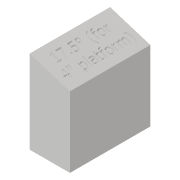
# Autodesk Inventor part: 20DegreeStand
Saved by Autodesk Inventor 2018 (Build 220112000, 112)
## iProperties
Created: 2018-12-13
Part Number: 20DegreeStand
Material: Generic
Document SubType Name: Modeling
Designer: ball
Density: 1 g/cm^3
Appearance: Default
Author: ball
Autodesk Inventor part; units mm, degrees
ref_plane "YZ Plane" through (0, 0, 0) normal (1, 0, 0) x (0, 1, 0)
ref_plane "XZ Plane" through (0, 0, 0) normal (0, 1, 0) x (-1, 0, 0)
ref_plane "XY Plane" through (0, 0, 0) normal (0, 0, 1) x (1, 0, 0)
sketch "Sketch1" plane through (0, 0, 0) normal (0, 1, 0) x (-1, 0, 0)
  line L0 (0, 0) -> (12.7, 0)
  line L1 (12.7, 0) -> (12.7, -25.4)
  line L2 (12.7, -25.4) -> (0, -25.4)
  line L3 (0, -25.4) -> (0, 0)
  dimension "d0" = 12.7
  dimension "d1" = 25.4
  constraints: 8 end point, 2 parallel, 1 horizontal, 1 perpendicular
  measures "d0" distance of L1.end L2.end
  measures "d1" distance of L0.end L1.end
extrude "Extrusion1" add sketch "Sketch1" along normal blind 26.289
sketch "Sketch2" plane through (-12.7, 0, 0) normal (0, 0, 1) x (1, 0, 0)
  line L0 (0, 0) -> (0, 26.289) projected
  line L1 (0, 26.289) -> (12.7, 26.289) projected
  line L2 (0, 26.289) -> (12.7, 26.289)
  line L3 (0, 26.289) -> (12.7, 22.2847)
  line L4 (0, 26.289) -> (13.3163, 26.289) construction
  line L5 (12.7, 0) -> (12.7, 26.289) projected
  line L6 (12.7, 22.2847) -> (12.7, 26.289)
  dimension "d4" = 17.5
  constraints: 8 end point, 1 collinear, 1 equal length, 1 horizontal, 1 perpendicular
  measures "d4" angle of L3 L4
extrude "Extrusion2" cut sketch "Sketch2" against normal blind 26.289
sketch "Sketch3" plane through (-12.7, 26.289, 0) normal (0.3007058, 0.953717, 0) x (0.953717, -0.3007058, 0)
  line L0 (2.3231, -6.9377) -> (2.3231, 32.6962) construction
  line L1 (2.3231, 32.6962) -> (11.3899, 32.6962) construction
  line L2 (11.3899, 32.6962) -> (11.3899, -6.9377) construction
  line L3 (11.3899, -6.9377) -> (2.3231, -6.9377) construction
  line L4 (5.5267, 5.1037) -> (5.5267, 3.6167)
  line L5 (5.5267, 3.6167) -> (5.2155, 3.6167)
  line L6 (5.2155, 3.6167) -> (5.2155, 4.17)
  line L7 (5.2155, 4.17) -> (3.1727, 4.17)
  line L8 (3.1727, 4.17) -> (3.1727, 3.6167)
  line L9 (3.1727, 3.6167) -> (2.8936, 3.6167)
  spline S0 degree 2 poles (2.8936, 3.6167) (2.8936, 3.9304) (2.7158, 4.2268) (2.4688, 4.2466) knots 0 0 0 1 2 2 2
  line L10 (2.4688, 4.2466) -> (2.4688, 4.5627)
  line L11 (2.4688, 4.5627) -> (5.2155, 4.5627)
  line L12 (5.2155, 4.5627) -> (5.2155, 5.1037)
  line L13 (5.2155, 5.1037) -> (5.5267, 5.1037)
  line L14 (2.9356, 7.5786) -> (5.5267, 6.2596)
  line L15 (5.5267, 6.2596) -> (5.5267, 5.8249)
  line L16 (5.5267, 5.8249) -> (2.8368, 7.218)
  line L17 (2.8368, 7.218) -> (2.8368, 5.6446)
  line L18 (2.8368, 5.6446) -> (2.4787, 5.6446)
  line L19 (2.4787, 5.6446) -> (2.4787, 7.5786)
  line L20 (2.4787, 7.5786) -> (2.9356, 7.5786)
  line L21 (5.5267, 8.6061) -> (5.5267, 8.1171)
  line L22 (5.5267, 8.1171) -> (4.9437, 8.1171)
  line L23 (4.9437, 8.1171) -> (4.9437, 8.6061)
  line L24 (4.9437, 8.6061) -> (5.5267, 8.6061)
  spline S1 degree 2 poles (4.5584, 11.0687) (4.7783, 11.0687) (5.1537, 10.928) (5.292, 10.7995) knots 0 0 0 1 2 2 2
  spline S2 degree 2 poles (5.292, 10.7995) (5.4303, 10.6711) (5.5909, 10.2882) (5.5909, 10.0511) knots 0 0 0 1 2 2 2
  spline S3 degree 2 poles (5.5909, 10.0511) (5.5909, 9.8337) (5.4946, 9.4089) (5.418, 9.2533) knots 0 0 0 1 2 2 2
  line L25 (5.418, 9.2533) -> (4.9857, 9.2533)
  line L26 (4.9857, 9.2533) -> (4.9857, 9.2829)
  spline S4 degree 2 poles (4.9857, 9.2829) (5.0203, 9.3299) (5.1092, 9.5052) (5.1488, 9.6114) knots 0 0 0 1 2 2 2
  spline S5 degree 2 poles (5.1488, 9.6114) (5.1907, 9.7325) (5.2377, 9.9325) (5.2377, 10.0585) knots 0 0 0 1 2 2 2
  spline S6 degree 2 poles (5.2377, 10.0585) (5.2377, 10.182) (5.1488, 10.4142) (5.0524, 10.4982) knots 0 0 0 1 2 2 2
  spline S7 degree 2 poles (5.0524, 10.4982) (4.961, 10.5747) (4.719, 10.6538) (4.556, 10.6538) knots 0 0 0 1 2 2 2
  spline S8 degree 2 poles (4.556, 10.6538) (4.3929, 10.6538) (4.1855, 10.5649) (4.1163, 10.4809) knots 0 0 0 1 2 2 2
  spline S9 degree 2 poles (4.1163, 10.4809) (4.0397, 10.3944) (3.9755, 10.1376) (3.9755, 9.9819) knots 0 0 0 1 2 2 2
  spline S10 degree 2 poles (3.9755, 9.9819) (3.9755, 9.814) (4.0274, 9.4805) (4.0496, 9.3793) knots 0 0 0 1 2 2 2
  line L27 (4.0496, 9.3793) -> (2.4787, 9.3793)
  line L28 (2.4787, 9.3793) -> (2.4787, 11.0515)
  line L29 (2.4787, 11.0515) -> (2.8368, 11.0515)
  line L30 (2.8368, 11.0515) -> (2.8368, 9.772)
  line L31 (2.8368, 9.772) -> (3.6495, 9.772)
  spline S11 degree 2 poles (3.6495, 9.772) (3.6396, 9.8461) (3.6322, 9.9894) (3.6322, 10.0486) knots 0 0 0 1 2 2 2
  spline S12 degree 2 poles (3.6322, 10.0486) (3.6322, 10.2833) (3.7087, 10.6069) (3.8224, 10.7551) knots 0 0 0 1 2 2 2
  spline S13 degree 2 poles (3.8224, 10.7551) (3.936, 10.9057) (4.2818, 11.0687) (4.5584, 11.0687) knots 0 0 0 1 2 2 2
  spline S14 degree 2 poles (3.2049, 13.0522) (3.5334, 13.0522) (3.9829, 12.6026) (3.9829, 12.2741) knots 0 0 0 1 2 2 2
  spline S15 degree 2 poles (3.9829, 12.2741) (3.9829, 11.9481) (3.5358, 11.4936) (3.2049, 11.4936) knots 0 0 0 1 2 2 2
  spline S16 degree 2 poles (3.2049, 11.4936) (2.8763, 11.4936) (2.4268, 11.9431) (2.4268, 12.2741) knots 0 0 0 1 2 2 2
  spline S17 degree 2 poles (2.4268, 12.2741) (2.4268, 12.6026) (2.8763, 13.0522) (3.2049, 13.0522) knots 0 0 0 1 2 2 2
  spline S18 degree 2 poles (3.2049, 12.7311) (3.0073, 12.7311) (2.738, 12.4692) (2.738, 12.2741) knots 0 0 0 1 2 2 2
  spline S19 degree 2 poles (2.738, 12.2741) (2.738, 12.0765) (3.0073, 11.8147) (3.2049, 11.8147) knots 0 0 0 1 2 2 2
  spline S20 degree 2 poles (3.2049, 11.8147) (3.4049, 11.8147) (3.6717, 12.0815) (3.6717, 12.2741) knots 0 0 0 1 2 2 2
  spline S21 degree 2 poles (3.6717, 12.2741) (3.6717, 12.4692) (3.4, 12.7311) (3.2049, 12.7311) knots 0 0 0 1 2 2 2
  line L32 (6.3689, 16.0211) -> (6.3689, 15.5518)
  spline S22 degree 2 poles (6.3689, 15.5518) (5.9466, 15.1961) (5.0006, 14.7886) (4.3559, 14.7886) knots 0 0 0 1 2 2 2
  spline S23 degree 2 poles (4.3559, 14.7886) (3.726, 14.7886) (2.7652, 15.1912) (2.3428, 15.5518) knots 0 0 0 1 2 2 2
  line L33 (2.3428, 15.5518) -> (2.3428, 16.0211)
  line L34 (2.3428, 16.0211) -> (2.3626, 16.0211)
  spline S24 degree 2 poles (2.3626, 16.0211) (2.5133, 15.8556) (2.9035, 15.5543) (3.1629, 15.4259) knots 0 0 0 1 2 2 2
  spline S25 degree 2 poles (3.1629, 15.4259) (3.4148, 15.3024) (4.02, 15.1492) (4.3559, 15.1492) knots 0 0 0 1 2 2 2
  spline S26 degree 2 poles (4.3559, 15.1492) (4.7066, 15.1492) (5.2871, 15.2974) (5.5489, 15.4259) knots 0 0 0 1 2 2 2
  spline S27 degree 2 poles (5.5489, 15.4259) (5.8008, 15.5494) (6.2084, 15.863) (6.3492, 16.0211) knots 0 0 0 1 2 2 2
  line L35 (6.3492, 16.0211) -> (6.3689, 16.0211)
  line L36 (2.7133, 17.6563) -> (2.7133, 17.6365)
  spline S28 degree 2 poles (2.7133, 17.6365) (2.6936, 17.5847) (2.659, 17.392) (2.659, 17.3154) knots 0 0 0 1 2 2 2
  spline S29 degree 2 poles (2.659, 17.3154) (2.659, 17.0734) (2.8763, 16.8659) (3.1629, 16.8659) knots 0 0 0 1 2 2 2
  line L37 (3.1629, 16.8659) -> (3.2394, 16.8659)
  line L38 (3.2394, 16.8659) -> (3.2394, 17.5031)
  line L39 (3.2394, 17.5031) -> (3.5581, 17.5031)
  line L40 (3.5581, 17.5031) -> (3.5581, 16.8782)
  line L41 (3.5581, 16.8782) -> (5.5267, 16.8782)
  line L42 (5.5267, 16.8782) -> (5.5267, 16.4929)
  line L43 (5.5267, 16.4929) -> (3.5581, 16.4929)
  line L44 (3.5581, 16.4929) -> (3.5581, 16.2336)
  line L45 (3.5581, 16.2336) -> (3.2394, 16.2336)
  line L46 (3.2394, 16.2336) -> (3.2394, 16.4929)
  line L47 (3.2394, 16.4929) -> (3.1629, 16.4929)
  spline S30 degree 2 poles (3.1629, 16.4929) (2.7528, 16.4929) (2.3231, 16.8906) (2.3231, 17.2611) knots 0 0 0 1 2 2 2
  spline S31 degree 2 poles (2.3231, 17.2611) (2.3231, 17.3673) (2.3453, 17.5723) (2.3601, 17.6563) knots 0 0 0 1 2 2 2
  line L48 (2.3601, 17.6563) -> (2.7133, 17.6563)
  spline S32 degree 2 poles (4.3831, 19.6669) (4.961, 19.6669) (5.5909, 19.1111) (5.5909, 18.6468) knots 0 0 0 1 2 2 2
  spline S33 degree 2 poles (5.5909, 18.6468) (5.5909, 18.17) (4.9413, 17.6242) (4.3831, 17.6242) knots 0 0 0 1 2 2 2
  spline S34 degree 2 poles (4.3831, 17.6242) (3.81, 17.6242) (3.1752, 18.1873) (3.1752, 18.6468) knots 0 0 0 1 2 2 2
  spline S35 degree 2 poles (3.1752, 18.6468) (3.1752, 19.1111) (3.8075, 19.6669) (4.3831, 19.6669) knots 0 0 0 1 2 2 2
  spline S36 degree 2 poles (4.3831, 19.2692) (3.9385, 19.2692) (3.5062, 18.9456) (3.5062, 18.6468) knots 0 0 0 1 2 2 2
  spline S37 degree 2 poles (3.5062, 18.6468) (3.5062, 18.3479) (3.9385, 18.0218) (4.3831, 18.0218) knots 0 0 0 1 2 2 2
  spline S38 degree 2 poles (4.3831, 18.0218) (4.8153, 18.0218) (5.2599, 18.3479) (5.2599, 18.6468) knots 0 0 0 1 2 2 2
  spline S39 degree 2 poles (5.2599, 18.6468) (5.2599, 18.9432) (4.8227, 19.2692) (4.3831, 19.2692) knots 0 0 0 1 2 2 2
  line L49 (3.6519, 21.2749) -> (3.6519, 21.2551)
  spline S40 degree 2 poles (3.6519, 21.2551) (3.6396, 21.2106) (3.6346, 21.1143) (3.6346, 21.0476) knots 0 0 0 1 2 2 2
  spline S41 degree 2 poles (3.6346, 21.0476) (3.6346, 20.892) (3.7705, 20.5857) (3.9039, 20.4474) knots 0 0 0 1 2 2 2
  line L50 (3.9039, 20.4474) -> (5.5267, 20.4474)
  line L51 (5.5267, 20.4474) -> (5.5267, 20.0621)
  line L52 (5.5267, 20.0621) -> (3.2394, 20.0621)
  line L53 (3.2394, 20.0621) -> (3.2394, 20.4474)
  line L54 (3.2394, 20.4474) -> (3.5803, 20.4474)
  spline S42 degree 2 poles (3.5803, 20.4474) (3.3926, 20.6574) (3.2394, 20.971) (3.2394, 21.1192) knots 0 0 0 1 2 2 2
  spline S43 degree 2 poles (3.2394, 21.1192) (3.2394, 21.1785) (3.2444, 21.2378) (3.2518, 21.2749) knots 0 0 0 1 2 2 2
  line L55 (3.2518, 21.2749) -> (3.6519, 21.2749)
  line L56 (9.4978, 3.8612) -> (9.4978, 3.4981)
  line L57 (9.4978, 3.4981) -> (10.5451, 3.4981)
  line L58 (10.5451, 3.4981) -> (10.5451, 3.1054)
  line L59 (10.5451, 3.1054) -> (9.4978, 3.1054)
  line L60 (9.4978, 3.1054) -> (9.4978, 1.7593)
  line L61 (9.4978, 1.7593) -> (9.0681, 1.7593)
  line L62 (9.0681, 1.7593) -> (7.4971, 3.1227)
  line L63 (7.4971, 3.1227) -> (7.4971, 3.4981)
  line L64 (7.4971, 3.4981) -> (9.1693, 3.4981)
  line L65 (9.1693, 3.4981) -> (9.1693, 3.8612)
  line L66 (9.1693, 3.8612) -> (9.4978, 3.8612)
  line L67 (9.1693, 3.1054) -> (7.9788, 3.1054)
  line L68 (7.9788, 3.1054) -> (9.1693, 2.0804)
  line L69 (9.1693, 2.0804) -> (9.1693, 3.1054)
  line L70 (7.3613, 4.6442) -> (8.5469, 4.5553)
  line L71 (8.5469, 4.5553) -> (8.5469, 4.2861)
  line L72 (8.5469, 4.2861) -> (7.3613, 4.1972)
  line L73 (7.3613, 4.1972) -> (7.3613, 4.6442)
  line L74 (7.3613, 5.4149) -> (8.5469, 5.326)
  line L75 (8.5469, 5.326) -> (8.5469, 5.0567)
  line L76 (8.5469, 5.0567) -> (7.3613, 4.9678)
  line L77 (7.3613, 4.9678) -> (7.3613, 5.4149)
  spline S44 degree 2 poles (9.3398, 9.152) (9.9128, 9.152) (10.5896, 8.6061) (10.5896, 8.1887) knots 0 0 0 1 2 2 2
  spline S45 degree 2 poles (10.5896, 8.1887) (10.5896, 8.0183) (10.5105, 7.7565) (10.429, 7.6206) knots 0 0 0 1 2 2 2
  line L78 (10.429, 7.6206) -> (11.3874, 7.6206)
  line L79 (11.3874, 7.6206) -> (11.3874, 7.2353)
  line L80 (11.3874, 7.2353) -> (8.2579, 7.2353)
  line L81 (8.2579, 7.2353) -> (8.2579, 7.6206)
  line L82 (8.2579, 7.6206) -> (8.4975, 7.6206)
  spline S46 degree 2 poles (8.4975, 7.6206) (8.3666, 7.7639) (8.1937, 8.1146) (8.1937, 8.3196) knots 0 0 0 1 2 2 2
  spline S47 degree 2 poles (8.1937, 8.3196) (8.1937, 8.7124) (8.8161, 9.152) (9.3398, 9.152) knots 0 0 0 1 2 2 2
  spline S48 degree 2 poles (9.3842, 8.7543) (8.9915, 8.7543) (8.5592, 8.5049) (8.5592, 8.2258) knots 0 0 0 1 2 2 2
  spline S49 degree 2 poles (8.5592, 8.2258) (8.5592, 8.0627) (8.705, 7.7565) (8.8186, 7.6206) knots 0 0 0 1 2 2 2
  line L83 (8.8186, 7.6206) -> (10.1178, 7.6206)
  spline S50 degree 2 poles (10.1178, 7.6206) (10.1894, 7.7713) (10.2438, 7.9862) (10.2438, 8.1245) knots 0 0 0 1 2 2 2
  spline S51 degree 2 poles (10.2438, 8.1245) (10.2438, 8.4234) (9.8041, 8.7543) (9.3842, 8.7543) knots 0 0 0 1 2 2 2
  line L84 (10.5451, 9.9449) -> (10.5451, 9.5596)
  line L85 (10.5451, 9.5596) -> (7.3613, 9.5596)
  line L86 (7.3613, 9.5596) -> (7.3613, 9.9449)
  line L87 (7.3613, 9.9449) -> (10.5451, 9.9449)
  spline S52 degree 2 poles (10.3031, 11.7851) (10.3376, 11.7381) (10.4611, 11.58) (10.4982, 11.5059) knots 0 0 0 1 2 2 2
  spline S53 degree 2 poles (10.4982, 11.5059) (10.5525, 11.4047) (10.6093, 11.2145) (10.6093, 11.0416) knots 0 0 0 1 2 2 2
  spline S54 degree 2 poles (10.6093, 11.0416) (10.6093, 10.9008) (10.5031, 10.6464) (10.4068, 10.55) knots 0 0 0 1 2 2 2
  spline S55 degree 2 poles (10.4068, 10.55) (10.3129, 10.4587) (10.0363, 10.3475) (9.8832, 10.3475) knots 0 0 0 1 2 2 2
  spline S56 degree 2 poles (9.8832, 10.3475) (9.646, 10.3475) (9.3101, 10.5476) (9.2138, 10.7649) knots 0 0 0 1 2 2 2
  spline S57 degree 2 poles (9.2138, 10.7649) (9.1249, 10.9576) (9.0582, 11.4812) (9.0409, 11.7851) knots 0 0 0 1 2 2 2
  line L88 (9.0409, 11.7851) -> (8.9668, 11.7851)
  spline S58 degree 2 poles (8.9668, 11.7851) (8.8334, 11.7851) (8.6679, 11.7035) (8.621, 11.6294) knots 0 0 0 1 2 2 2
  spline S59 degree 2 poles (8.621, 11.6294) (8.5741, 11.5553) (8.5444, 11.3429) (8.5444, 11.2293) knots 0 0 0 1 2 2 2
  spline S60 degree 2 poles (8.5444, 11.2293) (8.5444, 11.0959) (8.6235, 10.7353) (8.7, 10.555) knots 0 0 0 1 2 2 2
  line L89 (8.7, 10.555) -> (8.7, 10.5328)
  line L90 (8.7, 10.5328) -> (8.3073, 10.5328)
  spline S61 degree 2 poles (8.3073, 10.5328) (8.2776, 10.639) (8.2035, 11.0366) (8.2035, 11.2318) knots 0 0 0 1 2 2 2
  spline S62 degree 2 poles (8.2035, 11.2318) (8.2035, 11.4689) (8.2776, 11.7925) (8.374, 11.9209) knots 0 0 0 1 2 2 2
  spline S63 degree 2 poles (8.374, 11.9209) (8.4678, 12.0469) (8.7667, 12.1704) (8.9816, 12.1704) knots 0 0 0 1 2 2 2
  line L91 (8.9816, 12.1704) -> (10.5451, 12.1704)
  line L92 (10.5451, 12.1704) -> (10.5451, 11.7851)
  line L93 (10.5451, 11.7851) -> (10.3031, 11.7851)
  line L94 (9.982, 11.7851) -> (9.3472, 11.7851)
  spline S64 degree 2 poles (9.3472, 11.7851) (9.3595, 11.6467) (9.4015, 11.2293) (9.441, 11.0984) knots 0 0 0 1 2 2 2
  spline S65 degree 2 poles (9.441, 11.0984) (9.488, 10.9452) (9.6831, 10.7452) (9.856, 10.7452) knots 0 0 0 1 2 2 2
  spline S66 degree 2 poles (9.856, 10.7452) (10.0536, 10.7452) (10.2537, 10.9675) (10.2537, 11.1799) knots 0 0 0 1 2 2 2
  spline S67 degree 2 poles (10.2537, 11.1799) (10.2537, 11.3602) (10.0981, 11.6566) (9.982, 11.7851) knots 0 0 0 1 2 2 2
  spline S68 degree 2 poles (10.5896, 13.4029) (10.5896, 13.0892) (10.2314, 12.736) (9.8436, 12.736) knots 0 0 0 1 2 2 2
  line L95 (9.8436, 12.736) -> (8.5765, 12.736)
  line L96 (8.5765, 12.736) -> (8.5765, 12.4767)
  line L97 (8.5765, 12.4767) -> (8.2579, 12.4767)
  line L98 (8.2579, 12.4767) -> (8.2579, 12.736)
  line L99 (8.2579, 12.736) -> (7.6009, 12.736)
  line L100 (7.6009, 12.736) -> (7.6009, 13.1213)
  line L101 (7.6009, 13.1213) -> (8.2579, 13.1213)
  line L102 (8.2579, 13.1213) -> (8.2579, 13.8302)
  line L103 (8.2579, 13.8302) -> (8.5765, 13.8302)
  line L104 (8.5765, 13.8302) -> (8.5765, 13.1213)
  line L105 (8.5765, 13.1213) -> (9.6658, 13.1213)
  spline S69 degree 2 poles (9.6658, 13.1213) (9.8387, 13.1213) (10.0289, 13.1337) (10.1104, 13.1757) knots 0 0 0 1 2 2 2
  spline S70 degree 2 poles (10.1104, 13.1757) (10.182, 13.2103) (10.2537, 13.3659) (10.2537, 13.4992) knots 0 0 0 1 2 2 2
  spline S71 degree 2 poles (10.2537, 13.4992) (10.2537, 13.5931) (10.1969, 13.7685) (10.1796, 13.808) knots 0 0 0 1 2 2 2
  line L106 (10.1796, 13.808) -> (10.1796, 13.8302)
  line L107 (10.1796, 13.8302) -> (10.5254, 13.8302)
  spline S72 degree 2 poles (10.5254, 13.8302) (10.555, 13.7215) (10.5896, 13.4992) (10.5896, 13.4029) knots 0 0 0 1 2 2 2
  line L108 (7.7318, 15.3172) -> (7.7318, 15.2974)
  spline S73 degree 2 poles (7.7318, 15.2974) (7.712, 15.2455) (7.6774, 15.0529) (7.6774, 14.9763) knots 0 0 0 1 2 2 2
  spline S74 degree 2 poles (7.6774, 14.9763) (7.6774, 14.7343) (7.8948, 14.5268) (8.1813, 14.5268) knots 0 0 0 1 2 2 2
  line L109 (8.1813, 14.5268) -> (8.2579, 14.5268)
  line L110 (8.2579, 14.5268) -> (8.2579, 15.164)
  line L111 (8.2579, 15.164) -> (8.5765, 15.164)
  line L112 (8.5765, 15.164) -> (8.5765, 14.5391)
  line L113 (8.5765, 14.5391) -> (10.5451, 14.5391)
  line L114 (10.5451, 14.5391) -> (10.5451, 14.1538)
  line L115 (10.5451, 14.1538) -> (8.5765, 14.1538)
  line L116 (8.5765, 14.1538) -> (8.5765, 13.8944)
  line L117 (8.5765, 13.8944) -> (8.2579, 13.8944)
  line L118 (8.2579, 13.8944) -> (8.2579, 14.1538)
  line L119 (8.2579, 14.1538) -> (8.1813, 14.1538)
  spline S75 degree 2 poles (8.1813, 14.1538) (7.7713, 14.1538) (7.3415, 14.5515) (7.3415, 14.922) knots 0 0 0 1 2 2 2
  spline S76 degree 2 poles (7.3415, 14.922) (7.3415, 15.0282) (7.3637, 15.2332) (7.3786, 15.3172) knots 0 0 0 1 2 2 2
  line L120 (7.3786, 15.3172) -> (7.7318, 15.3172)
  spline S77 degree 2 poles (9.4015, 17.3278) (9.9795, 17.3278) (10.6093, 16.772) (10.6093, 16.3077) knots 0 0 0 1 2 2 2
  spline S78 degree 2 poles (10.6093, 16.3077) (10.6093, 15.8309) (9.9597, 15.2851) (9.4015, 15.2851) knots 0 0 0 1 2 2 2
  spline S79 degree 2 poles (9.4015, 15.2851) (8.8285, 15.2851) (8.1937, 15.8482) (8.1937, 16.3077) knots 0 0 0 1 2 2 2
  spline S80 degree 2 poles (8.1937, 16.3077) (8.1937, 16.772) (8.826, 17.3278) (9.4015, 17.3278) knots 0 0 0 1 2 2 2
  spline S81 degree 2 poles (9.4015, 16.9301) (8.9569, 16.9301) (8.5247, 16.6065) (8.5247, 16.3077) knots 0 0 0 1 2 2 2
  spline S82 degree 2 poles (8.5247, 16.3077) (8.5247, 16.0088) (8.9569, 15.6827) (9.4015, 15.6827) knots 0 0 0 1 2 2 2
  spline S83 degree 2 poles (9.4015, 15.6827) (9.8338, 15.6827) (10.2784, 16.0088) (10.2784, 16.3077) knots 0 0 0 1 2 2 2
  spline S84 degree 2 poles (10.2784, 16.3077) (10.2784, 16.6041) (9.8412, 16.9301) (9.4015, 16.9301) knots 0 0 0 1 2 2 2
  line L121 (8.6704, 18.9357) -> (8.6704, 18.916)
  spline S85 degree 2 poles (8.6704, 18.916) (8.658, 18.8715) (8.6531, 18.7752) (8.6531, 18.7085) knots 0 0 0 1 2 2 2
  spline S86 degree 2 poles (8.6531, 18.7085) (8.6531, 18.5529) (8.7889, 18.2466) (8.9223, 18.1083) knots 0 0 0 1 2 2 2
  line L122 (8.9223, 18.1083) -> (10.5451, 18.1083)
  line L123 (10.5451, 18.1083) -> (10.5451, 17.723)
  line L124 (10.5451, 17.723) -> (8.2579, 17.723)
  line L125 (8.2579, 17.723) -> (8.2579, 18.1083)
  line L126 (8.2579, 18.1083) -> (8.5988, 18.1083)
  spline S87 degree 2 poles (8.5988, 18.1083) (8.411, 18.3182) (8.2579, 18.6319) (8.2579, 18.7801) knots 0 0 0 1 2 2 2
  spline S88 degree 2 poles (8.2579, 18.7801) (8.2579, 18.8394) (8.2628, 18.8987) (8.2702, 18.9357) knots 0 0 0 1 2 2 2
  line L127 (8.2702, 18.9357) -> (8.6704, 18.9357)
  line L128 (10.5451, 21.8281) -> (9.2212, 21.8281)
  spline S89 degree 2 poles (9.2212, 21.8281) (9.0631, 21.8281) (8.7939, 21.8034) (8.7198, 21.7639) knots 0 0 0 1 2 2 2
  spline S90 degree 2 poles (8.7198, 21.7639) (8.6383, 21.7244) (8.5592, 21.5737) (8.5592, 21.4428) knots 0 0 0 1 2 2 2
  spline S91 degree 2 poles (8.5592, 21.4428) (8.5592, 21.3243) (8.705, 21.0526) (8.8433, 20.9093) knots 0 0 0 1 2 2 2
  spline S92 degree 2 poles (8.8433, 20.9093) (8.8779, 20.9118) (8.9742, 20.9167) (9.0384, 20.9167) knots 0 0 0 1 2 2 2
  line L129 (9.0384, 20.9167) -> (10.5451, 20.9167)
  line L130 (10.5451, 20.9167) -> (10.5451, 20.5314)
  line L131 (10.5451, 20.5314) -> (9.2212, 20.5314)
  spline S93 degree 2 poles (9.2212, 20.5314) (9.0631, 20.5314) (8.7939, 20.5067) (8.7198, 20.4672) knots 0 0 0 1 2 2 2
  spline S94 degree 2 poles (8.7198, 20.4672) (8.6383, 20.4276) (8.5592, 20.277) (8.5592, 20.1461) knots 0 0 0 1 2 2 2
  spline S95 degree 2 poles (8.5592, 20.1461) (8.5592, 20.0226) (8.7148, 19.7484) (8.8359, 19.6199) knots 0 0 0 1 2 2 2
  line L132 (8.8359, 19.6199) -> (10.5451, 19.6199)
  line L133 (10.5451, 19.6199) -> (10.5451, 19.2346)
  line L134 (10.5451, 19.2346) -> (8.2579, 19.2346)
  line L135 (8.2579, 19.2346) -> (8.2579, 19.6199)
  line L136 (8.2579, 19.6199) -> (8.5098, 19.6199)
  spline S96 degree 2 poles (8.5098, 19.6199) (8.3592, 19.7706) (8.1937, 20.067) (8.1937, 20.2449) knots 0 0 0 1 2 2 2
  spline S97 degree 2 poles (8.1937, 20.2449) (8.1937, 20.4474) (8.3789, 20.7611) (8.5889, 20.8426) knots 0 0 0 1 2 2 2
  spline S98 degree 2 poles (8.5889, 20.8426) (8.3937, 21.018) (8.1937, 21.349) (8.1937, 21.5416) knots 0 0 0 1 2 2 2
  spline S99 degree 2 poles (8.1937, 21.5416) (8.1937, 21.6898) (8.2851, 21.9319) (8.3888, 22.0208) knots 0 0 0 1 2 2 2
  spline S100 degree 2 poles (8.3888, 22.0208) (8.4925, 22.1122) (8.8038, 22.2135) (9.0384, 22.2135) knots 0 0 0 1 2 2 2
  line L137 (9.0384, 22.2135) -> (10.5451, 22.2135)
  line L138 (10.5451, 22.2135) -> (10.5451, 21.8281)
  spline S101 degree 2 poles (9.3743, 23.861) (10.0067, 23.861) (10.965, 23.4559) (11.3874, 23.0977) knots 0 0 0 1 2 2 2
  line L139 (11.3874, 23.0977) -> (11.3874, 22.6284)
  line L140 (11.3874, 22.6284) -> (11.3676, 22.6284)
  spline S102 degree 2 poles (11.3676, 22.6284) (11.2268, 22.7865) (10.8144, 23.1051) (10.5674, 23.2237) knots 0 0 0 1 2 2 2
  spline S103 degree 2 poles (10.5674, 23.2237) (10.3031, 23.3521) (9.7152, 23.5003) (9.3743, 23.5003) knots 0 0 0 1 2 2 2
  spline S104 degree 2 poles (9.3743, 23.5003) (9.0359, 23.5003) (8.4357, 23.3497) (8.1813, 23.2237) knots 0 0 0 1 2 2 2
  spline S105 degree 2 poles (8.1813, 23.2237) (7.9269, 23.1002) (7.5218, 22.784) (7.381, 22.6284) knots 0 0 0 1 2 2 2
  line L141 (7.381, 22.6284) -> (7.3613, 22.6284)
  line L142 (7.3613, 22.6284) -> (7.3613, 23.0977)
  spline S106 degree 2 poles (7.3613, 23.0977) (7.7836, 23.4534) (8.7371, 23.861) (9.3743, 23.861) knots 0 0 0 1 2 2 2
  point P0 (20.0175, 0)
  constraints: 2 other
emboss "Emboss1" sketch "Sketch3" operation cut depth 1.016 direction (-0.3007058, -0.953717, 0)
body "Solid1"
